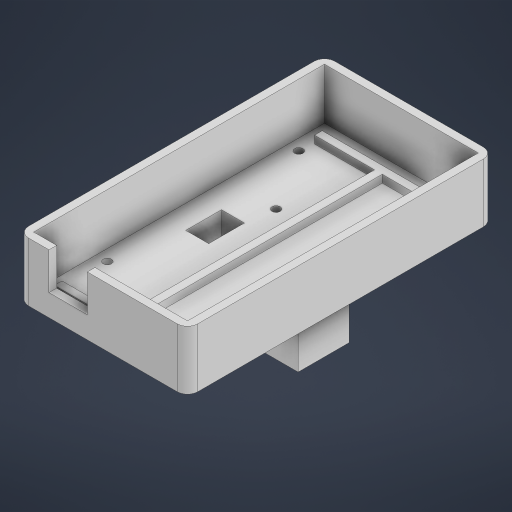
# Autodesk Inventor part: front_box
Saved by Autodesk Inventor 2024 (Build 280153000, 153)
## iProperties
Created: 2023-05-08
Part Number: front_box
Material: Типовые
Document SubType Name: Modeling
Designer: user
Density: 1 g/cm^3
Appearance: По умолчанию
Author: user
Autodesk Inventor part; units mm, degrees
ref_plane "YZ Plane" through (0, 0, 0) normal (1, 0, 0) x (0, 1, 0)
ref_plane "XZ Plane" through (0, 0, 0) normal (0, 1, 0) x (-1, 0, 0)
ref_plane "XY Plane" through (0, 0, 0) normal (0, 0, 1) x (1, 0, 0)
sketch "Эскиз1" plane through (0, 0, 0) normal (0, 0, 1) x (1, 0, 0)
  line L0 (20, 0) -> (35, 0)
  line L1 (35, 0) -> (35, -20)
  line L2 (35, -20) -> (20, -20)
  line L3 (20, -20) -> (20, 0)
  line L4 (0, -20) -> (90, -20) construction
  line L5 (0, 0) -> (90, 0) construction
  line L6 (35, -286) -> (35, 126) construction
  line L7 (55, -286) -> (55, 126) construction
  line L8 (70, -20) -> (55, -20)
  line L9 (55, -20) -> (55, 0)
  line L10 (55, 0) -> (70, 0)
  line L11 (70, 0) -> (70, -20)
  circle A0 centre (27.5, -10) radius 1.5
  circle A1 centre (62.5, -10) radius 1.5
  point P0 (62.5, -20)
  point P1 (27.5, -20)
  point P2 (70, -10)
  point P3 (20, -10)
  dimension "d0" = 15
  dimension "d1" = 15
  dimension "d2" = 3
  constraints: 16 end point, 5 point on line, 4 midpoint, 4 parallel, 3 vertical alignment, 2 centre point, 2 horizontal, 2 horizontal alignment, 2 perpendicular, 1 equal radius
  measures "d0" distance of L0.end L0.start
  measures "d1" distance of L9.end L10.end
  measures "d2" diameter of A1
ref_plane "РабПлоскость1" through (35, -286, 20) normal (0, 0, 1) x (1, 0, 0)
extrude "Выдавливание1" add sketch "Эскиз1" along normal up to surface (20 mm away)
sketch "Эскиз2" plane through (20, -20, 20) normal (0, 0, 1) x (1, 0, 0)
  line L0 (3, 3) -> (12, 3)
  line L1 (12, 3) -> (12, 17)
  line L2 (12, 17) -> (3, 17)
  line L3 (3, 17) -> (3, 3)
  line L4 (47, 3) -> (38, 3)
  line L5 (38, 3) -> (38, 17)
  line L6 (38, 17) -> (47, 17)
  line L7 (47, 17) -> (47, 3)
  line L8 (0, 0) -> (0, 20) projected
  line L9 (15, 0) -> (0, 0) projected
  line L10 (50, 0) -> (35, 0) projected
  point P0 (-20, 20)
  point P1 (3, 10)
  point P2 (0, 10)
  point P3 (38, 10)
  point P4 (12, 10)
  point P5 (7.5, 3)
  point P6 (7.5, 0)
  point P7 (42.5, 3)
  point P8 (42.5, 0)
  dimension "d5" = 3
  dimension "d6" = 3
  dimension "d7" = 3
  constraints: 16 end point, 8 midpoint, 4 parallel, 2 horizontal, 2 horizontal alignment, 2 perpendicular, 2 vertical alignment, 1 point on line
  measures "d5" horizontal distance of L8.start L0.start
  measures "d6" horizontal distance of L8.start L0.start
  measures "d7" horizontal distance of L10.end L4.end
extrude "Выдавливание2" cut sketch "Эскиз2" against normal blind 17
sketch "Эскиз3" plane through (55, 0, 20) normal (0, 0, 1) x (1, 0, 0)
  line L0 (22.0284, 49.4711) -> (-44.1693, 49.4711)
  line L1 (-44.1693, 49.4711) -> (-44.1693, -70.3219)
  line L2 (-44.1693, -70.3219) -> (22.0284, -70.3219)
  line L3 (22.0284, -70.3219) -> (22.0284, 49.4711)
  line L4 (3, -3) -> (12, -3) projected
  line L5 (3, -17) -> (3, -3) projected
  line L6 (12, -17) -> (3, -17) projected
  line L7 (12, -3) -> (12, -17) projected
  line L8 (-23, -3) -> (-23, -17) projected
  line L9 (-23, -17) -> (-32, -17) projected
  line L10 (-32, -17) -> (-32, -3) projected
  line L11 (-32, -3) -> (-23, -3) projected
  point P0 (-55, 0)
  constraints: 8 end point, 2 parallel, 1 horizontal, 1 perpendicular
extrude "Выдавливание3" add sketch "Эскиз3" along normal blind 3
sketch "Эскиз4" plane through (55, 0, 23) normal (0, 0, 1) x (1, 0, 0)
  line L0 (22.0284, -70.3219) -> (22.0284, 49.4711) projected
  line L1 (-44.1693, 49.4711) -> (-44.1693, -70.3219) projected
  line L2 (22.0284, 49.4711) -> (-44.1693, 49.4711)
  line L3 (-44.1693, 49.4711) -> (-44.1693, -70.3219)
  line L4 (-44.1693, -70.3219) -> (22.0284, -70.3219)
  line L5 (22.0284, -70.3219) -> (22.0284, 49.4711)
  line L6 (19.0284, 46.4711) -> (-41.1693, 46.4711)
  line L7 (-41.1693, 46.4711) -> (-41.1693, -67.3219)
  line L8 (-41.1693, -67.3219) -> (19.0284, -67.3219)
  line L9 (19.0284, -67.3219) -> (19.0284, 46.4711)
  point P0 (-55, 0)
  point P1 (-11.0704, -67.3219)
  point P2 (-11.0704, -70.3219)
  point P3 (19.0284, -10.4254)
  point P4 (22.0284, -10.4254)
  point P5 (-44.1693, 49.4711)
  dimension "d14" = 3
  dimension "d15" = 3
  constraints: 16 end point, 4 midpoint, 4 parallel, 2 horizontal, 2 perpendicular, 1 horizontal alignment, 1 vertical alignment
  measures "d14" horizontal distance of L0.start L8.end
  measures "d15" horizontal distance of L0.start L8.end
extrude "Выдавливание4" add sketch "Эскиз4" along normal blind 20
fillet "Сопряжение3" radius 4 4 edges at (77.0284, 49.4711, 31.5) (10.8307, 49.4711, 31.5) (10.8307, -70.3219, 31.5) (77.0284, -70.3219, 31.5)
sketch "Эскиз9" plane through (55, 0, 23) normal (0, 0, 1) x (1, 0, 0)
  line L0 (-36.0704, 40.4711) -> (13.9296, 40.4711)
  line L1 (13.9296, 40.4711) -> (13.9296, 37.4711)
  line L2 (-36.0704, 40.4711) -> (-36.0704, 37.4711)
  line L3 (-36.0704, 37.4711) -> (-12.5704, 37.4711)
  line L4 (-12.5704, 37.4711) -> (-12.5704, -61.3219)
  line L5 (-12.5704, -61.3219) -> (-36.0704, -61.3219)
  line L6 (-36.0704, -61.3219) -> (-36.0704, -64.3219)
  line L7 (-36.0704, -64.3219) -> (13.9296, -64.3219)
  line L8 (13.9296, -64.3219) -> (13.9296, -61.3219)
  line L9 (13.9296, -61.3219) -> (-9.5704, -61.3219)
  line L10 (-9.5704, -61.3219) -> (-9.5704, 37.4711)
  line L11 (-9.5704, 37.4711) -> (13.9296, 37.4711)
  line L12 (-41.1693, 46.4711) -> (19.0284, 46.4711) projected
  line L13 (19.0284, -67.3219) -> (-41.1693, -67.3219) projected
  point P0 (-55, 0)
  point P1 (-11.0704, 40.4711)
  point P2 (-11.0704, 46.4711)
  dimension "d20" = 3
  dimension "d21" = 6
  dimension "d22" = 50
  dimension "d23" = 3
  dimension "d24" = 50
  dimension "d25" = 6
  constraints: 24 end point, 9 perpendicular, 3 collinear, 2 horizontal, 2 horizontal alignment, 2 midpoint, 1 vertical, 1 vertical alignment
  measures "d20" distance of L10.end L3.end
  measures "d21" distance from line of L12 L0.start
  measures "d22" distance of L0.start L0.end
  measures "d23" distance of L0.start L2.end
  measures "d24" distance of L8.end L5.end
  measures "d25" distance from line of L8.end L13
extrude "Выдавливание5" add sketch "Эскиз9" along normal blind 3
sketch "Эскиз10" plane through (55, 0, 23) normal (0, 0, 1) x (1, 0, 0)
  circle A0 centre (11.4884, 38.3911) radius 1.636 projected
  circle A1 centre (6.4084, 7.9111) radius 1.636 projected
  circle A2 centre (-21.5316, 7.9111) radius 1.636 projected
  circle A3 centre (-36.7716, 32.0411) radius 1.636 projected
  circle A4 centre (-36.7716, -42.8889) radius 1.636 projected
  circle A5 centre (11.4884, -44.1589) radius 1.636 projected
  point P0 (-55, 0)
extrude "Выдавливание6" cut sketch "Эскиз10" against normal through all
move faces "Перенос1" translate (0, 0, 3.75) faces at (66.0268, 38.3008, 23)
sketch "Эскиз11" plane through (13.8307, -67.3219, 23) normal (0, 1, 0) x (1, 0, 0)
  line L0 (24, -20) -> (9, -20)
  line L1 (60.1977, -20) -> (0, -20) projected
  line L2 (9, -20) -> (9, -5.5)
  line L3 (9, -5.5) -> (24, -5.5)
  line L4 (24, -5.5) -> (24, -20)
  point P0 (-13.8307, 23)
  point P1 (16.5, -20)
  dimension "d34" = 15
  dimension "d36" = 9
  dimension "d39" = 14.5
  constraints: 8 end point, 2 horizontal, 1 midpoint, 1 parallel, 1 point on line, 1 vertical
  measures "d34" distance of L0.start L0.end
  measures "d36" distance of L1.end L0.end
  measures "d39" distance of L3.end L0.start
extrude "Выдавливание7" cut sketch "Эскиз11" against normal blind 10
sketch "Эскиз13" plane through (55, 0, 43) normal (0, 0, 1) x (1, 0, 0)
  circle A0 centre (8.0284, -74.3219) radius 2
  line L0 (12.0284, -80.3219) -> (4.0284, -80.3219) projected
  line L1 (14.0284, -70.3219) -> (14.0284, -78.3219) projected
  point P0 (-55, 0)
  point P1 (8.0284, -80.3219)
  point P2 (14.0284, -74.3219)
  dimension "d46" = 4
  constraints: 2 midpoint, 1 centre point, 1 horizontal alignment, 1 vertical alignment
  measures "d46" diameter of A0
extrude "Выдавливание9" cut sketch "Эскиз13" against normal through all
equation "\"d1\" = d0"
equation "\"d7\" = d6"
equation "\"d24\" = d22"
equation "\"d25\" = d21"
